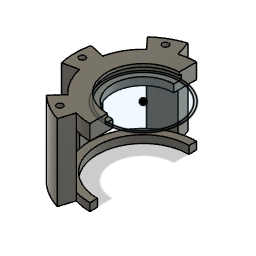
lamp holder v5 (Autodesk Fusion 360 design; units mm, degrees)
Autodesk Fusion 360 part; units mm, degrees
sketch "Skizze1" plane through (0, 0, 0) normal (0, 1, 0) x (1, 0, 0)
  circle A0 centre (0, 0) radius 35
  circle A1 centre (0, 0) radius 30
  circle A2 centre (0, 0) radius 45
  line L0 (0, 0) -> (0, 53) construction
  circle A3 centre (-20, 34.641) radius 2
  circle A4 centre (-40, 0) radius 2
  circle A5 centre (-20, -34.641) radius 2
  circle A6 centre (20, -34.641) radius 2
  circle A7 centre (40, 0) radius 2
  circle A8 centre (20, 34.641) radius 2
  line L1 (0, 0) -> (-30.4016, 33.1775)
  line L2 (-13.5318, 42.9173) -> (0, 0)
  line L3 (-20, 34.641) -> (0, 0) construction
  line L4 (-43.9333, 9.7398) -> (0, 0)
  line L5 (0, 0) -> (-43.9333, -9.7398)
  line L6 (-30.4016, -33.1775) -> (0, 0)
  line L7 (0, 0) -> (-13.5318, -42.9173)
  line L8 (13.5318, -42.9173) -> (0, 0)
  line L9 (0, 0) -> (30.4016, -33.1775)
  line L10 (43.9333, -9.7398) -> (0, 0)
  line L11 (0, 0) -> (43.9333, 9.7398)
  line L12 (30.4016, 33.1775) -> (0, 0)
  line L13 (0, 0) -> (13.5318, 42.9173)
  point P0 (-20, 34.641)
  point P1 (-40, 0)
  point P2 (-20, -34.641)
  point P3 (20, -34.641)
  point P4 (40, 0)
  point P5 (20, 34.641)
  dimension "d1" = 70
  dimension "d2" = 60
  dimension "d3" = 90
  dimension "d21" = 40
  dimension "d23" = 360
  dimension "d24" = 4
  dimension "d26" = 360
  dimension "d29" = 25
  dimension "d31" = 360
  constraint coincident A0.centre A1.centre
  constraint concentric A0 A1
  constraint concentric A1 A2
  constraint vertical L0
  constraint symmetric P0 P5 L0
  constraint coincident P0 A3.centre
  constraint coincident A2 L1.end
  constraint coincident A2 L2.start
  constraint symmetric L1 L2 L3
  measures "d1" diameter of A0
  measures "d2" diameter of A1
  measures "d3" diameter of A2
  measures "d21" distance of A0.centre P0
  measures "d24" diameter of A3
  measures "d29" angle of L1 L2
extrude "Extrusion1" add sketch "Skizze1" against normal blind 5 contours A0 A1 L10 L11 | A0 A2 L10 L11 | A0 A1 L11 L12 | A0 A2 L11 L12 | A0 A2 L9 L10 | A0 A1 L9 L10 | A0 A1 L12 L13 | A0 A2 L12 L13 | A0 A2 L8 L9 | A0 A1 L8 L9 | A0 A1 L2 L13 | A0 A2 L2 L13 | A0 A2 L7 L8 | A0 A1 L7 L8 | A0 A1 L1 L2 | A0 A2 L1 L2 | A0 A1 L1 L4 | A0 A1 L4 L5 | A0 A1 L5 L6 | A0 A1 L6 L7 | A0 A2 L6 L7 | A0 A2 L1 L4 | A0 A2 L4 L5 | A0 A2 L5 L6 | A3 | A4 | A5 | A6 | A7 | A8 makes body 1
extrude "Extrusion2" add sketch "Skizze1" along normal blind 35 contours A0 A2 L10 L11 | A0 A2 L11 L12 | A0 A2 L9 L10 | A0 A2 L12 L13 | A0 A2 L8 L9 | A0 A2 L2 L13 | A0 A2 L7 L8 | A0 A2 L1 L2 | A0 A2 L6 L7 | A0 A2 L1 L4 | A0 A2 L4 L5 | A0 A2 L5 L6 | A3 | A4 | A5 | A6 | A7 | A8 bodies 1
ref_plane "Arbeitsebene1" through (0, 35, 0) normal (0, 1, 0) x (0, 0, 1)
sketch "Skizze2" plane through (0, 35, 0) normal (0, 1, 0) x (1, 0, 0)
  circle A0 centre (0, 0) radius 20
  circle A1 centre (0, 0) radius 45
  circle A2 centre (0, 0) radius 23.5
  dimension "d9" = 40
  dimension "d10" = 90
  dimension "d11" = 47
  constraint coincident A0.centre A1.centre
  measures "d9" diameter of A0
  measures "d10" diameter of A1
  measures "d11" diameter of A2
extrude "Extrusion3" add sketch "Skizze2" along normal blind 10 contours A1 | A2 bodies 1
ref_plane "Arbeitsebene2" through (0, 40, 0) normal (0, 1, 0) x (0, 0, 1)
sketch "Skizze4" plane through (0, 40, 0) normal (0, 1, 0) x (1, 0, 0)
  circle A0 centre (0, 0) radius 23.5
  circle A1 centre (0, 0) radius 25
  dimension "d15" = 47
  dimension "d16" = 50
  constraint coincident A0.centre A1.centre
  constraint concentric A0 A1
  measures "d15" diameter of A0
  measures "d16" diameter of A1
extrude "Extrusion4" cut sketch "Skizze4" along normal through all contours A0 bodies 1
extrude "Extrusion5" cut sketch "Skizze4" along normal blind 3 contours A0 | A1 bodies 1
split "Teilen1" by plane through (0, 0, 0) normal (1, 0, 0) bodies 1 makes body 2 at (4.2775, 28.3333, -44.7962)
extrude "Extrusion6" cut sketch "Skizze1" along normal through all and the other way through all contours A3 | A4 | A5 | A6 | A7 | A8 bodies 1 2
extrude "Extrusion7" cut sketch "Skizze1" along normal through all and the other way through all contours A0 A2 L11 L12 | A0 A2 L9 L10 | A0 A2 L2 L13 | A0 A2 L7 L8 | A0 A2 L1 L4 | A0 A2 L5 L6 bodies 1 2
hidden bodies 2
